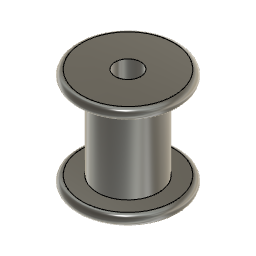
Roulette 1 v5 (archive) (Autodesk Fusion 360 design; units mm, degrees)
Autodesk Fusion 360 part; units mm, degrees
sketch "Esquisse1" plane through (0, 0, 0) normal (0, 0, 1) x (1, 0, 0)
  circle A0 centre (0, 0) radius 5
  dimension "d1" = 10
  constraint coincident A0.centre origin
  measures "d1" diameter of A0
extrude "Extrusion1" add sketch "Esquisse1" along normal blind 1
sketch "Esquisse2" plane through (0, 0, 1) normal (0, 0, 1) x (-1, 0, 0)
  circle A0 centre (0, 0) radius 5
  circle A1 centre (0, 0) radius 3
  dimension "d4" = 6
  constraint coincident A0.centre A1.centre
  measures "d4" diameter of A1
extrude "Extrusion2" add sketch "Esquisse2" along normal blind 8 contours A1
sketch "Esquisse3" plane through (0, 0, 9) normal (0, 0, 1) x (-1, 0, 0)
  circle A0 centre (0, 0) radius 3
  circle A1 centre (0, 0) radius 5
  dimension "d7" = 10
  constraint coincident A0.centre A1.centre
  measures "d7" diameter of A1
extrude "Extrusion3" add sketch "Esquisse3" along normal blind 1 contours A0 | A1
sketch "Esquisse4" plane through (0, 0, 10) normal (0, 0, 1) x (-1, 0, 0)
  circle A0 centre (0, 0) radius 5
  circle A1 centre (0, 0) radius 1.25
  dimension "d10" = 2.5
  constraint coincident A0.centre A1.centre
  measures "d10" diameter of A1
extrude "Extrusion4" cut sketch "Esquisse4" against normal blind 10 contours A1
fillet "Congé1" radius 0.5 4 edges at (-4.6616, -1.8081, 1) (4.6616, 1.8081, 9) (4.6616, 1.8081, 10) (-4.6616, -1.8081, 0)
